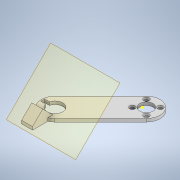
# Autodesk Inventor part: Pièce_moteur_maintient_test_7
Saved by Autodesk Inventor 2020.1 (Build 241239000, 239)
## iProperties
Created: 2019-07-26
Part Number: Pièce_moteur_maintient_test_7
Material: Générique
Document SubType Name: Modeling
Designer: marlo
Density: 1 g/cm^3
Appearance: Par défaut
Author: marlo
Autodesk Inventor part; units mm, degrees
ref_plane "YZ Plane" through (0, 0, 0) normal (1, 0, 0) x (0, 1, 0)
ref_plane "XZ Plane" through (0, 0, 0) normal (0, 1, 0) x (-1, 0, 0)
ref_plane "XY Plane" through (0, 0, 0) normal (0, 0, 1) x (1, 0, 0)
sketch "Esquisse3" plane through (0, 0, 0) normal (0, 1, 0) x (-1, 0, 0)
  line L0 (-9.2084, 3.7916) -> (3.7916, 3.7916) construction
  line L1 (3.7916, 3.7916) -> (3.7916, -9.2084) construction
  line L2 (3.7916, -9.2084) -> (-9.2084, -9.2084) construction
  line L3 (-9.2084, -9.2084) -> (-9.2084, 3.7916) construction
  line L4 (-9.2084, 3.7916) -> (3.7916, -9.2084) construction
  line L5 (3.7916, 3.7916) -> (-9.2084, -9.2084) construction
  line L6 (-14.2084, 8.7916) -> (8.7916, 8.7916) construction
  line L7 (8.7916, 8.7916) -> (8.7916, -14.2084) construction
  line L8 (8.7916, -14.2084) -> (-14.2084, -14.2084) construction
  line L9 (-14.2084, -14.2084) -> (-14.2084, 8.7916) construction
  line L10 (-14.2084, 8.7916) -> (8.7916, -14.2084) construction
  line L11 (8.7916, 8.7916) -> (-14.2084, -14.2084) construction
  line L12 (-9.2084, 3.7916) -> (-14.2084, 3.7916) construction
  line L13 (-14.2084, 3.7916) -> (-14.2084, 8.7916) construction
  line L14 (-14.2084, 8.7916) -> (-9.2084, 8.7916) construction
  line L15 (-9.2084, 8.7916) -> (-9.2084, 3.7916) construction
  line L16 (-9.2084, -9.2084) -> (-14.2084, -9.2084) construction
  line L17 (-14.2084, -9.2084) -> (-14.2084, -14.2084) construction
  line L18 (-14.2084, -14.2084) -> (-9.2084, -14.2084) construction
  line L19 (-9.2084, -14.2084) -> (-9.2084, -9.2084) construction
  line L20 (3.7916, -9.2084) -> (8.7916, -9.2084) construction
  line L21 (8.7916, -9.2084) -> (8.7916, -14.2084) construction
  line L22 (8.7916, -14.2084) -> (3.7916, -14.2084) construction
  line L23 (3.7916, -14.2084) -> (3.7916, -9.2084) construction
  line L24 (8.7916, 8.7916) -> (3.7916, 8.7916) construction
  line L25 (3.7916, 8.7916) -> (3.7916, 3.7916) construction
  line L26 (3.7916, 3.7916) -> (8.7916, 3.7916) construction
  line L27 (8.7916, 3.7916) -> (8.7916, 8.7916) construction
  circle A0 centre (6.2916, 6.2916) radius 2.5
  circle A1 centre (6.2916, -11.7084) radius 2.5
  circle A2 centre (-11.7084, -11.7084) radius 2.5
  circle A3 centre (-11.7084, 6.2916) radius 2.5
  circle A4 centre (-2.7084, -2.7084) radius 17.5
  circle A5 centre (-2.7084, -2.7084) radius 8.5
  circle A6 centre (55.9815, 55.9815) radius 17.5
  circle A7 centre (55.9815, 55.9815) radius 10
  line L28 (57.9815, 65.7795) -> (53.9815, 65.7795)
  line L29 (53.9815, 65.7795) -> (53.9815, 86.7795)
  line L30 (53.9815, 86.7795) -> (57.9815, 86.7795)
  line L31 (57.9815, 86.7795) -> (57.9815, 65.7795)
  line L32 (48.9815, 91.7795) -> (48.9815, 60.7795)
  line L33 (48.9815, 60.7795) -> (62.9815, 60.7795)
  line L34 (62.9815, 60.7795) -> (62.9815, 91.7795)
  line L35 (62.9815, 91.7795) -> (48.9815, 91.7795)
  line L36 (71.664, 53.4815) -> (65.664, 53.4815)
  line L37 (65.664, 53.4815) -> (65.664, 58.4815)
  line L38 (65.664, 58.4815) -> (71.664, 58.4815)
  line L39 (71.664, 58.4815) -> (71.664, 53.4815)
  line L40 (9.666, -15.0827) -> (-15.0827, 9.666) construction
  line L41 (9.666, -15.0827) -> (68.3559, 43.6071)
  line L42 (-15.0827, 9.666) -> (43.6071, 68.3559)
  line L43 (-15.0827, -15.0827) -> (68.3559, 68.3559) construction
  point P0 (6.2916, 6.2916)
  point P1 (73.4815, 55.9815)
  point P2 (17.4356, 66.5)
  point P3 (62.9815, 72.0205)
  point P4 (48.9815, 72.0205)
  point P5 (57.9815, 73.3668)
  point P6 (53.9815, 73.3668)
  point P7 (48.9815, 63.1229)
  point P8 (62.9815, 63.1229)
  dimension "d1" = 13
  dimension "d2" = 13
  dimension "d3" = 5
  dimension "d4" = 35
  dimension "d9" = 9
  dimension "d31" = 35
  dimension "d32" = 20
  dimension "d33" = 4
  dimension "d34" = 21
  dimension "d36" = 5
  dimension "d37" = 5
  dimension "d51" = 6
  dimension "d56" = 118
  constraints: 88 end point, 20 parallel, 12 tangent, 11 point on circle, 9 perpendicular, 8 centre point, 8 horizontal, 6 coincident, 4 collinear, 2 midpoint, 2 point on line, 3 other
  measures "d1" distance of L0.end L1.end
  measures "d2" distance of L0.start L0.end
  measures "d3" distance between parallel lines of L2 L8
  measures "d4" diameter of A4
  measures "d9" radial gap between concentric circles of A4 A5
  measures "d31" diameter of A6
  measures "d32" diameter of A7
  measures "d33" distance of L29.end L30.end
  measures "d34" distance of L30.end L28.start
  measures "d36" distance between parallel lines of L29 L32
  measures "d37" distance of L38.end L36.start
  measures "d51" distance of L36.start L36.end
  measures "d56" distance of L43.start L43.end
extrude "Extrusion1" add sketch "Esquisse3" along normal blind 4 contours A4 | A4 L42 A6 L41 | A6 L32 A7 L36 L39 L38 L34 | L32 L35 L34 A6 L31 L30 L29 | A6 L29 A7 L32 | L34 A7 L31 A6
chamfer "Chanfrein5" distance 1 distance2 2 1 edges at (14.2084, 4, -11.7084) measured on face at (14.7084, 4, -11.7084)
chamfer "Chanfrein6" distance 1 distance2 2 1 edges at (-3.7916, 4, -11.7084) measured on face at (-3.2916, 4, -11.7084)
chamfer "Chanfrein7" distance 1 distance2 2 1 edges at (-3.7916, 4, 6.2916) measured on face at (-3.2916, 4, 6.2916)
chamfer "Chanfrein8" distance 1 distance2 2 1 edges at (14.2084, 4, 6.2916) measured on face at (14.7084, 4, 6.2916)
ref_plane "Plan de construction1" through (-62.9815, 4, 91.7795) normal (0, 0.7071068, 0.7071068) x (1, 0, 0)
sketch "Esquisse8" plane through (-62.9815, 4, 91.7795) normal (0, 0.7071068, 0.7071068) x (1, 0, 0)
  line L0 (0, 11.1433) -> (0, -2.8284) projected
  line L1 (0, 0) -> (14, 0)
  line L2 (14, 0) -> (14, 18.3465)
  line L3 (14, 18.3465) -> (0, 18.3465)
  line L4 (0, 18.3465) -> (0, 0)
  line L5 (9, 3.5355) -> (5, 3.5355) projected
  line L6 (9, 3.5355) -> (5, 3.5355)
  line L7 (5, 3.5355) -> (5, 18.3465)
  line L8 (5, 18.3465) -> (9, 18.3465)
  line L9 (9, 18.3465) -> (9, 3.5355)
  line L10 (14, 0) -> (14, 13.9717) projected
  line L11 (5, 3.5355) -> (5, 18.3848) projected
  point P0 (62.9815, 62.0694)
  point P1 (9, 18.3465)
  point P2 (5, 3.5355)
  constraints: 16 end point, 4 parallel, 2 collinear, 2 horizontal, 2 perpendicular, 2 point on line
extrude "Extrusion3" add sketch "Esquisse8" against normal up to surface contours L4 L3 L7 L5 L9 L2 L1 L0 surface through (2.7084, 4, -2.7084) normal (0, 1, 0)
sketch "Esquisse9" plane through (-53.9815, 6.5, 89.2795) normal (0, 0.7071068, -0.7071068) x (-1, 0, 0)
  line L0 (0, -3.5355) -> (4, -3.5355) projected
  line L1 (0, -3.5355) -> (4, -3.5355)
  line L2 (4, -3.5355) -> (4, 0)
  line L3 (4, 0) -> (0, 0)
  line L4 (0, 0) -> (0, -3.5355)
  line L5 (4, 0) -> (4, -18.3465) projected
  point P0 (-53.9815, -67.7263)
  constraints: 8 end point, 2 parallel, 1 collinear, 1 horizontal, 1 perpendicular
extrude "Extrusion4" add sketch "Esquisse9" along normal up to surface (14.811 mm away)
sketch "Esquisse10" plane through (0, 4, 0) normal (0, 1, 0) x (1, 0, 0)
  point P0 (0, 0)
